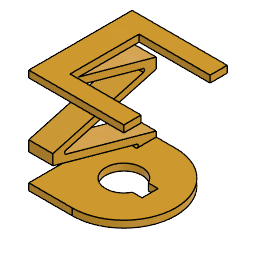
キースイッチ-サンプル (Autodesk Fusion 360 archive; units mm, degrees)
design "ボタン-スプリング"
Autodesk Fusion 360 part; units mm, degrees
note: some values were not read from the file. Set by a fixed rule: which face or edge a step refers to.
sketch "スケッチ1" plane through (0, 0, 0) normal (0, 0, 1) x (1, 0, 0)
  circle A0 centre (0, 0) radius 2.65
  line L0 (0, -7.5) -> (0, 7.5)
  line L1 (0, 7.5) -> (-6.3, 7.5)
  line L2 (-6.3, 7.5) -> (-6.3, -7.5)
  line L3 (-6.3, -7.5) -> (0, -7.5)
  line L4 (0, -7.5) -> (0, 7.5)
  arc A1 (0, -7.5) -> (0, 7.5) centre (0, 0) ccw
  line L5 (2.65, 0) -> (-2.65, 0)
  line L6 (3.8, 1.15) -> (1.5, 1.15)
  line L7 (1.5, 1.15) -> (1.5, -1.15)
  line L8 (1.5, -1.15) -> (3.8, -1.15)
  line L9 (3.8, -1.15) -> (3.8, 1.15)
  line L10 (3.8, 1.15) -> (1.5, -1.15) construction
  line L11 (1.5, 1.15) -> (3.8, -1.15) construction
  point P0 (2.65, 0)
  dimension "d1" = 5.3
  dimension "d2" = 15
  dimension "d5" = 6.3
  dimension "d6" = 15
  dimension "d31" = 2.3
  dimension "d32" = 2.3
  constraint coincident A0.centre A1.centre
  constraint midpoint L0 A0.centre
  constraint vertical L0
  constraint horizontal L1
  constraint vertical L2
  constraint horizontal L3
  constraint vertical L4
  constraint midpoint L5 A0.centre
  constraint coincident A0 L5.end
  constraint perpendicular L0 L5
  constraint horizontal L6
  constraint perpendicular L6 L7
  constraint parallel L6 L8
  constraint parallel L7 L9
  constraint coincident L10 P0
  constraint coincident L11 P0
  constraint coincident P0 L5.start
  measures "d1" diameter of A0
  measures "d2" diameter of A1
  measures "d5" distance of A0.centre L2
  measures "d6" distance of L1 L3
  measures "d31" distance of L7.end L8.end
  measures "d32" distance of L6.end L7.end
extrude "押し出し1" add sketch "スケッチ1" along normal blind 1 contours A0 L0 L4 A1 L6 L8 L9 | A0 L0 L1 L2 L3 L4
sketch "スケッチ2" plane through (-6.3, 0, 0) normal (-1, 0, 0) x (0, -1, 0)
  line L0 (-7.5, 0) -> (7.5, 0)
  line L1 (7.5, 0) -> (7.5, 1)
  line L2 (7.5, 1) -> (-7.5, 1)
  line L3 (-7.5, 1) -> (-7.5, 0)
  line L4 (-7.5, 1) -> (-7.5, 16) construction
  line L5 (7.5, 1) -> (7.5, 16) construction
  line L6 (-7.5, 1) -> (-7.5, 1.7604)
  line L7 (-6.5, 1) -> (-7.5, 1)
  line L8 (-7.5, 1) -> (-7.5, 1.7604)
  line L9 (-4.7298, 1.4909) -> (7.5, 4.8825)
  line L10 (-4.663, 1) -> (10.2045, 1) construction
  line L11 (-7.5, 1.7604) -> (5.6313, 5.4021)
  line L12 (5.6313, 5.8839) -> (-7.5, 9.5255)
  line L13 (-5.6313, 10.045) -> (7.5, 6.4034)
  line L14 (7.5, 6.4034) -> (7.5, 4.8825)
  line L15 (-5.6313, 10.5268) -> (7.5, 14.1685)
  line L16 (-7.5, 11.0463) -> (3.758, 14.1685)
  line L17 (-7.5, 11.0463) -> (-7.5, 9.5255)
  line L18 (7.5, 14.1685) -> (3.758, 14.1685)
  arc A0 (-4.7298, 1.4909) -> (-4.663, 1) centre (-4.663, 1.25) ccw
  arc A1 (5.6313, 5.4021) -> (5.6313, 5.8839) centre (5.5645, 5.643) ccw
  arc A2 (-5.6313, 10.5268) -> (-5.6313, 10.045) centre (-5.5645, 10.2859) ccw
  point P0 (6.5, 5.643)
  point P1 (-6.5, 10.2859)
  dimension "d7" = 15
  dimension "d8" = 15
  dimension "d9" = 15.5
  dimension "d15" = 15.5
  dimension "d16" = 1
  dimension "d17" = 1
  dimension "d18" = 15.5
  dimension "d19" = 15.5
  dimension "d20" = 1
  dimension "d21" = 1
  dimension "d22" = 15.5
  dimension "d23" = 15.5
  dimension "d24" = 1
  dimension "d25" = 1
  dimension "d26" = 0.25
  dimension "d27" = 0.25
  dimension "d28" = 0.25
  constraint coincident L2.end L3.start
  constraint perpendicular L2 L4
  constraint coincident L1.end L2.start
  constraint perpendicular L2 L5
  constraint coincident L4 L6.end
  constraint horizontal L7
  constraint vertical L8
  constraint coincident L2 L7.start
  constraint horizontal L10
  constraint coincident L5 L9.end
  constraint coincident L5 L13.end
  constraint coincident L4 L12.end
  constraint coincident L4 L16.start
  constraint coincident L5 L15.end
  constraint parallel L10 L18
  constraint coincident L7.start L9
  constraint coincident L7.start L10
  constraint tangent L9 A0
  constraint tangent L10 A0
  constraint coincident P0 L11
  constraint coincident P0 L12
  constraint tangent L11 A1
  constraint tangent L12 A1
  constraint coincident P1 L15
  constraint coincident P1 L13
  constraint tangent L15 A2
  constraint tangent L13 A2
  measures "d7" distance of L2.end L4.end
  measures "d8" distance of L1.end L5.end
  measures "d9" angle of L9 L10
  measures "d15" angle of L10 L11
  measures "d16" distance of L9 L11
  measures "d17" distance of L7.start L2.end
  measures "d18" angle of L10 L12
  measures "d19" angle of L10 L13
  measures "d20" distance of L12 L13
  measures "d21" distance of P0 L14
  measures "d22" angle of L10 L15
  measures "d23" angle of L10 L16
  measures "d24" distance of L15 L16
  measures "d25" distance of P1 L17
  measures "d26" radius of A0
  measures "d27" radius of A1
  measures "d28" radius of A2
extrude "押し出し2" add sketch "スケッチ2" against normal blind 3.5 contours L2 L6 L7 L8 L9 L11 L12 L13 L14 L15 L16 L17 L18 A0 A1 A2
sketch "スケッチ3" plane through (0, 0, 14.1685) normal (0, 0, 1) x (-1, 0, 0)
  line L0 (6.3, 3.758) -> (6.3, 7.5)
  line L1 (6.3, 7.5) -> (2.8, 7.5)
  line L2 (2.8, 7.5) -> (2.8, 3.758)
  line L3 (2.8, 3.758) -> (6.3, 3.758)
  line L4 (2.8, -4.663) -> (6.3, -4.663)
  line L5 (6.3, -4.663) -> (6.3, 7.5)
  line L6 (6.3, 7.5) -> (0, 7.5)
  arc A0 (0, 7.5) -> (0, -7.5) centre (0, 0) ccw
  line L7 (0, -7.5) -> (2.8, -7.5)
  line L8 (2.8, -7.5) -> (2.8, -4.663)
  line L9 (-3.8, -1.15) -> (-3.8, 1.15)
  line L10 (-3.8, 1.15) -> (-2.3875, 1.15)
  arc A1 (-2.3875, -1.15) -> (-2.3875, 1.15) centre (0, 0) ccw
  line L11 (-2.3875, -1.15) -> (-3.8, -1.15)
  line L12 (6.3, -7.5) -> (6.3, 3.758)
  line L13 (6.3, 3.758) -> (2.8, 3.758)
  line L14 (2.8, 3.758) -> (2.8, -7.5)
  line L15 (2.8, -7.5) -> (6.3, -7.5)
  line L16 (6.3, 5) -> (6.3, -5)
  line L17 (-7.5, 0) -> (-7.5, -7.5)
  line L18 (-7.5, -7.5) -> (6.3, -7.5)
  line L19 (6.3, -4.663) -> (6.3, -7.5)
  line L20 (6.3, -5) -> (-7.5, -5)
  line L21 (-20, 0) -> (-2.5, 0)
  line L22 (6.3, 5) -> (-7.5, 5)
  line L23 (-7.5, 0) -> (-7.5, 7.5)
  line L24 (6.3, 4.663) -> (6.3, 7.5)
  line L25 (-7.5, 7.5) -> (6.3, 7.5)
  point P0 (6.3, 0)
  dimension "d38" = 5
  constraint midpoint L16 P0
  constraint coincident L12 P0
  constraint coincident L12 L16.end
  constraint midpoint A0 L17.start
  constraint tangent A0 L17
  constraint perpendicular L7 L17
  constraint coincident L12.start L15.end
  constraint perpendicular L12 L18
  constraint coincident L4.end L5.start
  constraint coincident L17 L20.end
  constraint perpendicular L17 L20
  constraint symmetric L17.start L21 L23.start
  constraint symmetric L17.end L21 L23.end
  constraint symmetric L12.start L21 L0.end
  constraint symmetric L4.end L21 L24.start
  constraint symmetric L16.end L21 L16.start
  constraint symmetric L20.end L21 L22.end
  measures "d38" distance of A0.centre L20
extrude "押し出し3" add sketch "スケッチ3" along normal blind 1 contours L0 L2 L3 L5 L13 L16 L22 L24 | L3 L4 L5 L12 L13 L14 L16 | L4 L8 L12 L14 L16 L19 L20 | L0 L1 L2 L5 L6 L22 L24 L25 | L2 L6 A0 L22 L25 | L8 L12 L14 L15 L18 L19 L20 | A0 L22 L23 L25 | A0 L7 L8 L14 L18 L20 | A0 L17 L18 L20
equation "d5 = d1 + 1 mm"
equation "d6 = d2"
equation "d8 = d7"
equation "d15 = d9"
equation "d17 = d16"
equation "d18 = d9"
equation "d19 = d9"
equation "d20 = d16"
equation "d21 = d16"
equation "d22 = d9"
equation "d23 = d9"
equation "d24 = d16"
equation "d25 = d16"
equation "d31 = d32"

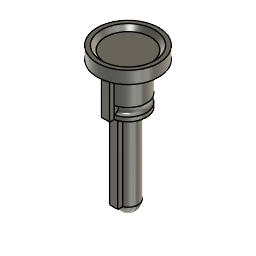
design "ボタンA"
Autodesk Fusion 360 part; units mm, degrees
sketch "スケッチ1" plane through (0, 0, 0) normal (0, 0, 1) x (1, 0, 0)
  circle A0 centre (0, 0) radius 7.5
  dimension "d1" = 15
  constraint coincident A0.centre origin
  measures "d1" diameter of A0
extrude "押し出し1" add sketch "スケッチ1" along normal blind 2
sketch "スケッチ2" plane through (0, 0, 2) normal (0, 0, 1) x (-1, 0, 0)
  circle A0 centre (0, 0) radius 7.5
  circle A1 centre (0, 0) radius 6.5
  dimension "d4" = 13
  constraint coincident A0.centre A1.centre
  measures "d4" diameter of A1
extrude "押し出し2" add sketch "スケッチ2" along normal blind 1
chamfer "面取り1" distance 1 angle 45 1 edges at (6.0601, 2.3505, 2)
sketch "スケッチ3" plane through (0, 0, 0) normal (0, 0, -1) x (1, 0, 0)
  circle A0 centre (0, 0) radius 7.5
  line L0 (0, -2.5) -> (0, 2.5)
  circle A1 centre (0, 0) radius 2.5
  line L1 (1, 1.5) -> (-1, 1.5)
  line L2 (-1, 1.5) -> (-1, 3.5)
  line L3 (-1, 3.5) -> (1, 3.5)
  line L4 (1, 3.5) -> (1, 1.5)
  line L5 (1, 1.5) -> (-1, 3.5) construction
  line L6 (-1, 1.5) -> (1, 3.5) construction
  circle A2 centre (0, 0) radius 4.5
  line L7 (0.9923, 5.5) -> (-1.0077, 5.5)
  line L8 (-1.0077, 5.5) -> (-1.0077, 3.5)
  line L9 (-1.0077, 3.5) -> (0.9923, 3.5)
  line L10 (0.9923, 3.5) -> (0.9923, 5.5)
  line L11 (0.9923, 5.5) -> (-1.0077, 3.5) construction
  line L12 (-1.0077, 5.5) -> (0.9923, 3.5) construction
  point P0 (0, 2.5)
  point P1 (0, 2.5)
  point P2 (-0.0077, 4.5)
  dimension "d8" = 5
  dimension "d15" = 2.5
  dimension "d22" = 2
  dimension "d23" = 2
  dimension "d24" = 9
  dimension "d25" = 2
  dimension "d26" = 2
  constraint coincident A0.centre A1.centre
  constraint midpoint L0 A0.centre
  constraint vertical L0
  constraint coincident P1 P0
  constraint horizontal L1
  constraint perpendicular L1 L2
  constraint parallel L1 L3
  constraint parallel L2 L4
  constraint coincident L5 P1
  constraint coincident L6 P1
  constraint horizontal L7
  constraint perpendicular L7 L8
  constraint parallel L7 L9
  constraint parallel L8 L10
  constraint coincident L11 P2
  constraint coincident L12 P2
  constraint coincident A2 P2
  measures "d8" diameter of A1
  measures "d15" distance of A0.centre P1
  measures "d22" distance of L2.end L3.end
  measures "d23" distance of L1.end L2.end
  measures "d24" diameter of A2
  measures "d25" distance of L7.end L8.end
  measures "d26" distance of L7.start L7.end
extrude "押し出し3" add sketch "スケッチ3" along normal blind 29.45 contours L0 A1 L1 L2 | L0 A1 L1 L4 | L0 A1 L1 L2 | L0 A1 L1 L4 | A1 L2 L3 L4 L9
sketch "スケッチ5" plane through (0, 0, 0) normal (0, 0, -1) x (1, 0, 0)
  line L0 (-1, 2.2913) -> (-1, 3.5)
  line L1 (-1, 3.5) -> (0.9923, 3.5)
  line L2 (1, 3.5) -> (1, 2.2913)
  arc A0 (-1, 2.2913) -> (1, 2.2913) centre (0, 0) ccw
  circle A1 centre (0, 0) radius 7.5
  line L3 (0.9923, 3.5) -> (1, 3.5)
extrude "押し出し4" add sketch "スケッチ3" along normal blind 10 contours A1 L2 L3 L4 A2 L8 L9 L10 | L3 A2 L8 L9 L10 | A2 L7 L8 L10
sphere "球プリミティブ1" add diameter 5 placed x (1, 0, 0) y (0, -1, 0) z (0, 0, -1) at (0, 0, -29.45)
ref_plane "作業平面1" through (0, 0, -8) normal (0, 0, 1) x (-1, 0, 0)
sketch "スケッチ7" plane through (0, 0, -8) normal (0, 0, 1) x (1, 0, 0)
  circle A0 centre (0, 0) radius 4.5
  arc A1 (0.9923, -4.3892) -> (-1.0077, -4.3857) centre (0, 0) ccw
  line L0 (0.9923, -4.3892) -> (0.9923, -5.5)
  line L1 (0.9923, -5.5) -> (-1.0077, -5.5)
  line L2 (-1.0077, -5.5) -> (-1.0077, -4.3857)
  line L3 (0.9923, -3.5) -> (1, -3.5)
  line L4 (1, -3.5) -> (1, -2.2913)
  arc A2 (1, -2.2913) -> (-1, -2.2913) centre (0, 0) ccw
  line L5 (-1, -2.2913) -> (-1, -3.5)
  line L6 (-1, -3.5) -> (0.9923, -3.5)
  line L7 (-1.0077, -5.5) -> (1, -5.5)
  line L8 (1, -5.5) -> (1, -3.5)
  line L9 (1, -3.5) -> (-1.0077, -3.5)
  line L10 (-1.0077, -3.5) -> (-1.0077, -5.5)
  line L11 (1, -2.2913) -> (-1, -2.2913)
  line L12 (-1, -2.2913) -> (-1, -3.5)
  line L13 (-1, -3.5) -> (1, -3.5)
  line L14 (1, -3.5) -> (1, -2.2913)
  dimension "d31" = 9
  constraint coincident A0.centre A1.centre
  constraint horizontal L7
  constraint vertical L8
  constraint horizontal L9
  constraint vertical L10
  constraint coincident L3.end L4.start
  constraint coincident L1.end L2.start
  constraint horizontal L11
  constraint vertical L12
  constraint horizontal L13
  constraint vertical L14
  constraint coincident L5.end L6.start
  constraint coincident L4.end A2.start
  measures "d31" diameter of A0
torus "トーラス プリミティブ1" cut centre line diameter 9 section diameter 2 placed x (1, 0, 0) y (0, 1, 0) z (0, 0, 1) at (0, 0, -8)
extrude "押し出し5" add sketch "スケッチ7" along normal blind 2 and the other way blind 1.9 contours A0 A1 L3 L6 L8 L9 L10 L13 | A0 L0 L1 L2 L7 L10 | L3 L4 L5 L6 L9 L11 L12 L13 L14
equation "d9 = 26 mm + 3.45 mm"
equation "d24 = d8 + 4 mm"

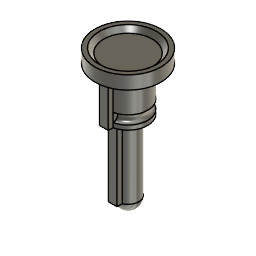
design "ボタンC"
Autodesk Fusion 360 part; units mm, degrees
sketch "スケッチ1" plane through (0, 0, 0) normal (0, 0, 1) x (1, 0, 0)
  circle A0 centre (0, 0) radius 7.5
  dimension "d1" = 15
  constraint coincident A0.centre origin
  measures "d1" diameter of A0
extrude "押し出し1" add sketch "スケッチ1" along normal blind 2
sketch "スケッチ2" plane through (0, 0, 2) normal (0, 0, 1) x (-1, 0, 0)
  circle A0 centre (0, 0) radius 7.5
  circle A1 centre (0, 0) radius 6.5
  dimension "d4" = 13
  constraint coincident A0.centre A1.centre
  measures "d4" diameter of A1
extrude "押し出し2" add sketch "スケッチ2" along normal blind 1
chamfer "面取り1" distance 1 angle 45 1 edges at (6.0601, 2.3505, 2)
sketch "スケッチ3" plane through (0, 0, 0) normal (0, 0, -1) x (1, 0, 0)
  circle A0 centre (0, 0) radius 7.5
  line L0 (0, -2.5) -> (0, 2.5)
  circle A1 centre (0, 0) radius 2.5
  line L1 (1, 1.5) -> (-1, 1.5)
  line L2 (-1, 1.5) -> (-1, 3.5)
  line L3 (-1, 3.5) -> (1, 3.5)
  line L4 (1, 3.5) -> (1, 1.5)
  line L5 (1, 1.5) -> (-1, 3.5) construction
  line L6 (-1, 1.5) -> (1, 3.5) construction
  circle A2 centre (0, 0) radius 4.5
  line L7 (0.9923, 5.5) -> (-1.0077, 5.5)
  line L8 (-1.0077, 5.5) -> (-1.0077, 3.5)
  line L9 (-1.0077, 3.5) -> (0.9923, 3.5)
  line L10 (0.9923, 3.5) -> (0.9923, 5.5)
  line L11 (0.9923, 5.5) -> (-1.0077, 3.5) construction
  line L12 (-1.0077, 5.5) -> (0.9923, 3.5) construction
  point P0 (0, 2.5)
  point P1 (0, 2.5)
  point P2 (-0.0077, 4.5)
  dimension "d8" = 5
  dimension "d15" = 2.5
  dimension "d22" = 2
  dimension "d23" = 2
  dimension "d24" = 9
  dimension "d25" = 2
  dimension "d26" = 2
  constraint coincident A0.centre A1.centre
  constraint midpoint L0 A0.centre
  constraint vertical L0
  constraint coincident P1 P0
  constraint horizontal L1
  constraint perpendicular L1 L2
  constraint parallel L1 L3
  constraint parallel L2 L4
  constraint coincident L5 P1
  constraint coincident L6 P1
  constraint horizontal L7
  constraint perpendicular L7 L8
  constraint parallel L7 L9
  constraint parallel L8 L10
  constraint coincident L11 P2
  constraint coincident L12 P2
  constraint coincident A2 P2
  measures "d8" diameter of A1
  measures "d15" distance of A0.centre P1
  measures "d22" distance of L2.end L3.end
  measures "d23" distance of L1.end L2.end
  measures "d24" diameter of A2
  measures "d25" distance of L7.end L8.end
  measures "d26" distance of L7.start L7.end
extrude "押し出し3" add sketch "スケッチ3" along normal blind 26 contours L0 A1 L1 L2 | L0 A1 L1 L4 | L0 A1 L1 L2 | L0 A1 L1 L4 | A1 L2 L3 L4 L9
sketch "スケッチ5" plane through (0, 0, 0) normal (0, 0, -1) x (1, 0, 0)
  line L0 (-1, 2.2913) -> (-1, 3.5)
  line L1 (-1, 3.5) -> (0.9923, 3.5)
  line L2 (1, 3.5) -> (1, 2.2913)
  arc A0 (-1, 2.2913) -> (1, 2.2913) centre (0, 0) ccw
  circle A1 centre (0, 0) radius 7.5
  line L3 (0.9923, 3.5) -> (1, 3.5)
extrude "押し出し4" add sketch "スケッチ3" along normal blind 10 contours A1 L2 L3 L4 A2 L8 L9 L10 | L3 A2 L8 L9 L10 | A2 L7 L8 L10
sphere "球プリミティブ1" add diameter 5 placed x (1, 0, 0) y (0, -1, 0) z (0, 0, -1) at (0, 0, -26)
ref_plane "作業平面1" through (0, 0, -8) normal (0, 0, 1) x (-1, 0, 0)
sketch "スケッチ7" plane through (0, 0, -8) normal (0, 0, 1) x (1, 0, 0)
  circle A0 centre (0, 0) radius 4.5
  arc A1 (0.9923, -4.3892) -> (-1.0077, -4.3857) centre (0, 0) ccw
  line L0 (0.9923, -4.3892) -> (0.9923, -5.5)
  line L1 (0.9923, -5.5) -> (-1.0077, -5.5)
  line L2 (-1.0077, -5.5) -> (-1.0077, -4.3857)
  line L3 (0.9923, -3.5) -> (1, -3.5)
  line L4 (1, -3.5) -> (1, -2.2913)
  arc A2 (1, -2.2913) -> (-1, -2.2913) centre (0, 0) ccw
  line L5 (-1, -2.2913) -> (-1, -3.5)
  line L6 (-1, -3.5) -> (0.9923, -3.5)
  line L7 (-1.0077, -5.5) -> (1, -5.5)
  line L8 (1, -5.5) -> (1, -3.5)
  line L9 (1, -3.5) -> (-1.0077, -3.5)
  line L10 (-1.0077, -3.5) -> (-1.0077, -5.5)
  line L11 (1, -2.2913) -> (-1, -2.2913)
  line L12 (-1, -2.2913) -> (-1, -3.5)
  line L13 (-1, -3.5) -> (1, -3.5)
  line L14 (1, -3.5) -> (1, -2.2913)
  dimension "d31" = 9
  constraint coincident A0.centre A1.centre
  constraint horizontal L7
  constraint vertical L8
  constraint horizontal L9
  constraint vertical L10
  constraint coincident L3.end L4.start
  constraint coincident L1.end L2.start
  constraint horizontal L11
  constraint vertical L12
  constraint horizontal L13
  constraint vertical L14
  constraint coincident L5.end L6.start
  constraint coincident L4.end A2.start
  measures "d31" diameter of A0
torus "トーラス プリミティブ1" cut centre line diameter 9 section diameter 2 placed x (1, 0, 0) y (0, 1, 0) z (0, 0, 1) at (0, 0, -8)
extrude "押し出し5" add sketch "スケッチ7" along normal blind 2 and the other way blind 1.9 contours A0 A1 L3 L6 L8 L9 L10 L13 | A0 L0 L1 L2 L7 L10 | L3 L4 L5 L6 L9 L11 L12 L13 L14
equation "d24 = d8 + 4 mm"

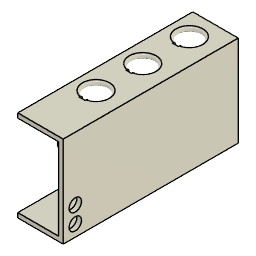
design "キースイッチ-サンプル土台"
Autodesk Fusion 360 part; units mm, degrees
sketch "スケッチ2" plane through (0, 0, 0) normal (0, 0, 1) x (1, 0, 0)
  line L0 (9, -65.0568) -> (9, 9.9432)
  line L1 (9, 9.9432) -> (-8.5, 9.9432)
  line L2 (-8.5, 9.9432) -> (-8.5, -65.0568)
  circle A0 centre (0, 0) radius 4.75
  line L3 (0, -4.75) -> (0, 4.75)
  line L4 (-1.25, -6) -> (1.25, -6)
  line L5 (1.25, -6) -> (1.25, -3.5)
  line L6 (1.25, -3.5) -> (-1.25, -3.5)
  line L7 (-1.25, -3.5) -> (-1.25, -6)
  line L8 (-1.25, -6) -> (1.25, -3.5) construction
  line L9 (1.25, -6) -> (-1.25, -3.5) construction
  line L10 (1.25, -23.5) -> (-1.25, -23.5)
  line L11 (1.25, -26) -> (1.25, -23.5)
  line L12 (0, -24.75) -> (0, -15.25)
  line L13 (-1.25, -26) -> (1.25, -26)
  line L14 (1.25, -26) -> (-1.25, -23.5) construction
  line L15 (-1.25, -23.5) -> (-1.25, -26)
  line L16 (-1.25, -26) -> (1.25, -23.5) construction
  circle A1 centre (0, -20) radius 4.75
  line L17 (1.25, -46) -> (-1.25, -43.5) construction
  line L18 (-1.25, -43.5) -> (-1.25, -46)
  line L19 (-1.25, -46) -> (1.25, -46)
  line L20 (0, -44.75) -> (0, -35.25)
  line L21 (1.25, -46) -> (1.25, -43.5)
  line L22 (1.25, -43.5) -> (-1.25, -43.5)
  circle A2 centre (0, -40) radius 4.75
  line L23 (-1.25, -46) -> (1.25, -43.5) construction
  line L24 (9, -65.0568) -> (-8.5, -65.0568)
  point P0 (0, -4.75)
  point P1 (0, -20)
  point P2 (0, -20)
  point P3 (0, -24.75)
  point P4 (0, -44.75)
  point P5 (0, -40)
  point P6 (0, -40)
  dimension "d4" = 9.5
  dimension "d5" = 2.5
  dimension "d6" = 2.5
  dimension "d16" = 9
  dimension "d17" = 8.5
  dimension "d48" = 9.5
  dimension "d49" = 2.5
  dimension "d50" = 2.5
  dimension "d51" = 20
  dimension "d55" = 9.5
  dimension "d56" = 2.5
  dimension "d57" = 2.5
  dimension "d61" = 20
  dimension "d108" = 75
  constraint parallel L0 L2
  constraint coincident A0.centre origin
  constraint coincident A0 P0
  constraint coincident A0 L3.end
  constraint vertical L3
  constraint horizontal L4
  constraint perpendicular L4 L5
  constraint parallel L4 L6
  constraint parallel L5 L7
  constraint coincident L8 P0
  constraint coincident L9 P0
  constraint coincident P0 L3.start
  constraint vertical A0.centre P0
  constraint coincident P2 P1
  constraint coincident P3 A1
  constraint coincident L12.end A1
  constraint vertical L12
  constraint horizontal L13
  constraint perpendicular L11 L13
  constraint parallel L10 L13
  constraint parallel L11 L15
  constraint coincident P3 L16
  constraint coincident P3 L14
  constraint coincident P3 L12.start
  constraint vertical P3 P2
  constraint coincident P6 P5
  constraint coincident P4 A2
  constraint coincident L20.end A2
  constraint vertical L20
  constraint horizontal L19
  constraint perpendicular L19 L21
  constraint parallel L19 L22
  constraint parallel L18 L21
  constraint coincident P4 L23
  constraint coincident P4 L17
  constraint coincident P4 L20.start
  constraint vertical P4 P6
  constraint vertical A0.centre P5
  constraint vertical A0.centre P2
  constraint horizontal L24
  constraint coincident L2.end L24.end
  constraint perpendicular L1 L2
  constraint perpendicular L2 L24
  measures "d4" diameter of A0
  measures "d5" distance of L5.end L6.end
  measures "d6" distance of L4.end L5.end
  measures "d16" distance of L0 A0.centre
  measures "d17" distance of L2 A0.centre
  measures "d48" diameter of A1
  measures "d49" distance of L10.start L10.end
  measures "d50" distance of L11.start L10.start
  measures "d51" distance of A0.centre P2
  measures "d55" diameter of A2
  measures "d56" distance of L21.end L17.end
  measures "d57" distance of L21.end L17.start
  measures "d61" distance of P2 P6
  measures "d108" distance of L0.start L0.end
extrude "押し出し2" add sketch "スケッチ2" along normal blind 2
sketch "スケッチ3" plane through (9, 0, 0) normal (1, 0, 0) x (0, 1, 0)
  line L0 (-65.0568, 0) -> (9.9432, 0)
  line L1 (9.9432, 0) -> (9.9432, 2)
  line L2 (9.9432, 2) -> (-65.0568, 2)
  line L3 (-65.0568, 2) -> (9.9432, 2)
  line L4 (9.9432, 2) -> (9.9432, -37)
  line L5 (9.9432, -37) -> (-65.0568, -37)
  line L6 (-65.0568, -37) -> (-65.0568, 2)
  line L7 (-65.0568, 2) -> (-65.0568, 0)
  point P0 (9.9432, 2)
  dimension "d11" = 39
  constraint horizontal L3
  constraint vertical L4
  constraint horizontal L5
  constraint vertical L6
  constraint coincident L2.end L3.start
  constraint coincident P0 L1.end
  measures "d11" distance of P0 L4.end
extrude "押し出し3" add sketch "スケッチ3" along normal blind 2
sketch "スケッチ4" plane through (9, 0, 0) normal (-1, 0, 0) x (0, -1, 0)
  line L0 (65.0568, 0) -> (-9.9432, 0)
  line L1 (-9.9432, 0) -> (-9.9432, -37)
  line L2 (-9.9432, -37) -> (65.0568, -37)
  line L3 (65.0568, -37) -> (65.0568, 0)
  line L4 (-9.9432, 0) -> (65.0568, 0)
  line L5 (-9.9432, -37) -> (65.0568, -37)
  line L6 (65.0568, -37) -> (65.0568, -35)
  line L7 (65.0568, -35) -> (-9.9432, -35)
  line L8 (-9.9432, -35) -> (-9.9432, -37)
  line L9 (48.0568, 0) -> (50.0568, 0)
  line L10 (48.0568, -17) -> (-9.9432, -17)
  line L11 (-9.9432, -17) -> (-9.9432, -19)
  line L12 (-9.9432, -19) -> (48.0568, -19)
  line L13 (48.0568, -17) -> (48.0568, -19)
  dimension "d47" = 2
  dimension "d111" = 2
  dimension "d112" = 17
  dimension "d135" = 58
  constraint horizontal L5
  constraint vertical L6
  constraint horizontal L7
  constraint vertical L8
  constraint coincident L3 L6.end
  constraint coincident L1.end L2.start
  constraint horizontal L9
  constraint coincident L0 L9.start
  constraint horizontal L10
  constraint vertical L11
  constraint horizontal L12
  constraint coincident L1 L11.end
  constraint perpendicular L12 L13
  constraint coincident L10.start L13.start
  measures "d47" distance of L2.end L6.end
  measures "d111" distance of L10 L12
  measures "d112" distance of L4 L10
  measures "d135" distance of L1 L13
extrude "押し出し4" add sketch "スケッチ4" along normal blind 17.5 contours L1 L2 L3 L5 L6 L7 L8 | L1 L10 L11 L12 L13
sketch "スケッチ5" plane through (0, 0, -17) normal (0, 0, 1) x (-1, 0, 0)
  line L0 (8.5, -9.9432) -> (8.5, 48.0568)
  line L1 (-9, 65.0568) -> (-9, 50.0568)
  line L2 (-9, -9.9432) -> (8.5, -9.9432)
  circle A0 centre (0, 0) radius 2.65
  line L3 (0, 2.65) -> (0, -2.65)
  line L4 (1.15, 4) -> (1.15, 1.5)
  line L5 (1.15, 1.5) -> (-1.15, 1.5)
  line L6 (-1.15, 1.5) -> (-1.15, 4)
  line L7 (3, 7) -> (-3, 7)
  line L8 (-3, 7) -> (-3, 4)
  line L9 (-3, 4) -> (3, 4)
  line L10 (3, 4) -> (3, 7)
  line L11 (3, 7) -> (-3, 4) construction
  line L12 (-3, 7) -> (3, 4) construction
  circle A1 centre (0, 20) radius 2.65
  line L13 (-3, 27) -> (3, 24) construction
  line L14 (-1.15, 21.5) -> (-1.15, 24)
  line L15 (0, 22.65) -> (0, 17.35)
  line L16 (-3, 27) -> (-3, 24)
  line L17 (1.15, 21.5) -> (-1.15, 21.5)
  line L18 (1.15, 24) -> (1.15, 21.5)
  line L19 (-3, 24) -> (3, 24)
  line L20 (3, 27) -> (-3, 24) construction
  line L21 (3, 24) -> (3, 27)
  line L22 (3, 27) -> (-3, 27)
  line L23 (-1.15, 41.5) -> (-1.15, 44)
  line L24 (1.15, 44) -> (1.15, 41.5)
  line L25 (-3, 47) -> (-3, 44)
  line L26 (1.15, 41.5) -> (-1.15, 41.5)
  line L27 (-3, 47) -> (3, 44) construction
  line L28 (3, 47) -> (-3, 44) construction
  line L29 (3, 47) -> (-3, 47)
  line L30 (0, 42.65) -> (0, 37.35)
  circle A2 centre (0, 40) radius 2.65
  line L31 (-3, 44) -> (3, 44)
  line L32 (3, 44) -> (3, 47)
  line L33 (-9, 50.0568) -> (8.5, 50.0568)
  line L34 (-9, 48.0568) -> (-9, -9.9432)
  line L35 (8.5, 48.0568) -> (-9, 48.0568)
  line L36 (-9, 48.0568) -> (-9, -9.9432)
  line L37 (-9, -9.9432) -> (8.5, -9.9432)
  line L38 (8.5, -9.9432) -> (8.5, 48.0568)
  line L39 (8.5, 48.0568) -> (-9, 48.0568)
  line L40 (-9, 48.0568) -> (-9, -9.9432)
  line L41 (-9, -9.9432) -> (8.5, -9.9432)
  line L42 (8.5, -9.9432) -> (8.5, 48.0568)
  line L43 (8.5, -9.9432) -> (-9, -9.9432)
  line L44 (-9, -9.9432) -> (-9, -6.4432)
  line L45 (-9, -6.4432) -> (8.5, -6.4432)
  line L46 (8.5, -6.4432) -> (8.5, -9.9432)
  line L47 (8.5, 13.5568) -> (-9, 13.5568)
  line L48 (-9, 13.5568) -> (-9, 11.5568)
  line L49 (-9, 11.5568) -> (8.5, 11.5568)
  line L50 (8.5, 11.5568) -> (8.5, 13.5568)
  line L51 (8.5, 33.5568) -> (-9, 33.5568)
  line L52 (-9, 33.5568) -> (-9, 31.5568)
  line L53 (-9, 31.5568) -> (8.5, 31.5568)
  line L54 (8.5, 31.5568) -> (8.5, 33.5568)
  line L55 (8.5, 48.0568) -> (-9, 48.0568)
  point P0 (0, 2.65)
  point P1 (0, 5.5)
  point P2 (0, 20)
  point P3 (0, 20)
  point P4 (0, 22.65)
  point P5 (0, 25.5)
  point P6 (0, 40)
  point P7 (0, 42.65)
  point P8 (0, 45.5)
  point P9 (0, 40)
  dimension "d22" = 5.3
  dimension "d23" = 2.3
  dimension "d87" = 6
  dimension "d88" = 3
  dimension "d89" = 5.5
  dimension "d90" = 1.5
  dimension "d91" = 2.3
  dimension "d92" = 5.3
  dimension "d93" = 2.3
  dimension "d94" = 6
  dimension "d95" = 3
  dimension "d96" = 5.5
  dimension "d97" = 1.5
  dimension "d98" = 2.3
  dimension "d99" = 20
  dimension "d100" = 5.3
  dimension "d101" = 2.3
  dimension "d102" = 6
  dimension "d103" = 3
  dimension "d104" = 5.5
  dimension "d105" = 1.5
  dimension "d106" = 2.3
  dimension "d107" = 20
  dimension "d116" = 3.5
  dimension "d117" = 20
  dimension "d118" = 2
  dimension "d119" = 20
  dimension "d120" = 2
  constraint coincident A0.centre origin
  constraint midpoint L3 A0.centre
  constraint coincident A0 L3.end
  constraint parallel L0 L3
  constraint parallel L4 L6
  constraint coincident P0 L3.start
  constraint horizontal L7
  constraint perpendicular L7 L8
  constraint parallel L7 L9
  constraint parallel L8 L10
  constraint coincident L11 P1
  constraint coincident L12 P1
  constraint coincident L4.start L9
  constraint perpendicular L4 L9
  constraint coincident L6.end L9
  constraint perpendicular L3 L5
  constraint coincident P3 P2
  constraint midpoint P3 L15
  constraint coincident L15.end A1
  constraint parallel L14 L18
  constraint coincident P4 L15.start
  constraint horizontal L22
  constraint perpendicular L16 L22
  constraint parallel L19 L22
  constraint parallel L16 L21
  constraint coincident P5 L20
  constraint coincident P5 L13
  constraint coincident L18.start L19
  constraint perpendicular L18 L19
  constraint coincident L14.end L19
  constraint perpendicular L15 L17
  constraint coincident P9 P6
  constraint midpoint P9 L30
  constraint coincident L30.end A2
  constraint parallel L23 L24
  constraint coincident P7 L30.start
  constraint horizontal L29
  constraint perpendicular L25 L29
  constraint parallel L29 L31
  constraint parallel L25 L32
  constraint coincident P8 L28
  constraint coincident P8 L27
  constraint coincident L24.start L31
  constraint perpendicular L24 L31
  constraint coincident L23.end L31
  constraint perpendicular L26 L30
  constraint vertical A0.centre P3
  constraint vertical A0.centre P9
  constraint vertical P5 P8
  constraint horizontal L43
  constraint vertical L44
  constraint horizontal L45
  constraint vertical L46
  constraint coincident L0.start L2.end
  constraint horizontal L47
  constraint vertical L48
  constraint horizontal L49
  constraint vertical L50
  constraint coincident L40 L48.end
  constraint coincident L0 L47.start
  constraint horizontal L51
  constraint vertical L52
  constraint horizontal L53
  constraint vertical L54
  constraint coincident L40 L52.end
  constraint coincident L38 L51.start
  measures "d22" diameter of A0
  measures "d23" distance of L4.end L5.end
  measures "d87" distance of L8.end L9.end
  measures "d88" distance of L7.end L8.end
  measures "d89" distance of A0.centre P1
  measures "d90" distance of A0.centre L5
  measures "d92" diameter of A1
  measures "d93" distance of L17.start L14.start
  measures "d94" distance of L16.end L13.end
  measures "d95" distance of L13.start L16.end
  measures "d96" distance of P3 P5
  measures "d97" distance of P3 L17
  measures "d99" distance of A0.centre P3
  measures "d100" diameter of A2
  measures "d101" distance of L23.start L24.end
  measures "d102" distance of L25.end L27.end
  measures "d103" distance of L25.start L25.end
  measures "d104" distance of P8 P9
  measures "d105" distance of P9 L26
  measures "d107" distance of P3 P9
  measures "d116" distance of L0.start L45.end
  measures "d117" distance of L45 L47
  measures "d118" distance of L47 L49
  measures "d119" distance of L47 L51
  measures "d120" distance of L51 L53
extrude "押し出し14" cut sketch "スケッチ5" along normal blind 2 from surface at -2 contours A0 L3 L4 L5 | A0 L3 L5 L6 | A0 L4 L6 L9 | A0 L3 L5 L6 | A0 L3 L4 L5 | L7 L8 L9 L10 | A1 L15 L17 L18 | A1 L14 L15 L17 | A1 L14 L18 L19 | A1 L14 L15 L17 | A1 L15 L17 L18 | L16 L19 L21 L22 | L23 L26 L30 A2 | L23 L26 L30 A2 | L23 L24 A2 L31 | L24 L26 L30 A2 | L24 L26 L30 A2 | L25 L29 L31 L32
extrude "押し出し15" add sketch "スケッチ5" along normal blind 1 contours L0 L2 L34 L36 L37 L38 L40 L41 L42 L43 L44 L45 L46 | L0 L34 L36 L38 L40 L42 L47 L48 L49 L50 | L0 L34 L36 L38 L40 L42 L51 L52 L53 L54
fillet "フィレット1" radius 1 12 edges at (0, 2.65, -17) (0, -17.35, -17) (0, -37.35, -17) (0, 4.75, 2) (0, -15.25, 2) (0, -35.25, 2) (0, -35.25, 0) (0, -15.25, 0) (0, 4.75, 0) (0, 2.65, -19) (0, -17.35, -19) (0, -37.35, -19)
sketch "スケッチ11" plane through (9, 0, 0) normal (-1, 0, 0) x (0, -1, 0)
  circle A0 centre (59.8875, -25) radius 2.5
  spline S0 degree 3 poles (43.4641, -17) (43.3309, -17) (43.1738, -17.0302) (42.9274, -17.128) (42.7936, -17.2125) (42.606, -17.3902) (42.5173, -17.5135) (42.4179, -17.7392) (42.3875, -17.88) (42.3875, -18) knots 0.151292 0.151292 0.151292 0.151292 0.191268 0.191268 0.230832 0.230832 0.268794 0.268794 0.304806 0.304806 0.304806 0.304806
  line L0 (36.35, -19) -> (43.4641, -19)
  spline S1 degree 3 poles (42.3875, -18) (42.3875, -17.88) (42.4179, -17.7392) (42.5173, -17.5135) (42.606, -17.3902) (42.7936, -17.2125) (42.9274, -17.128) (43.1738, -17.0302) (43.3309, -17) (43.4641, -17) knots 0.304806 0.304806 0.304806 0.304806 0.340818 0.340818 0.37878 0.37878 0.418344 0.418344 0.45832 0.45832 0.45832 0.45832
  line L1 (37.3875, -17) -> (42.3875, -17)
  line L2 (42.3875, -17) -> (42.3875, -18)
  line L3 (42.3875, -18) -> (37.3875, -18)
  line L4 (37.3875, -18) -> (37.3875, -17)
  line L5 (39.8875, -21.7117) -> (39.8875, -12.2883)
  circle A1 centre (59.8875, -32) radius 2.5
  line L6 (43.4641, -17) -> (36.35, -17)
  spline S2 degree 3 poles (42.3875, -18) (42.3875, -18.12) (42.4179, -18.2608) (42.5173, -18.4865) (42.606, -18.6098) (42.7936, -18.7875) (42.9274, -18.872) (43.1738, -18.9698) (43.3309, -19) (43.4641, -19) knots 0.304806 0.304806 0.304806 0.304806 0.340818 0.340818 0.37878 0.37878 0.418344 0.418344 0.45832 0.45832 0.45832 0.45832
  spline S3 degree 3 poles (43.4641, -19) (43.3309, -19) (43.1738, -18.9698) (42.9274, -18.872) (42.7936, -18.7875) (42.606, -18.6098) (42.5173, -18.4865) (42.4179, -18.2608) (42.3875, -18.12) (42.3875, -18) knots 0.151292 0.151292 0.151292 0.151292 0.191268 0.191268 0.230832 0.230832 0.268794 0.268794 0.304806 0.304806 0.304806 0.304806
  point P0 (39.8875, -17)
  dimension "d125" = 5
  dimension "d126" = 20
  dimension "d127" = 6
  dimension "d131" = 5
  dimension "d132" = 5
  dimension "d133" = 7
  constraint horizontal L1
  constraint vertical L2
  constraint horizontal L3
  constraint vertical L4
  constraint coincident S0.end S1.start
  constraint midpoint L5 P0
  constraint coincident L1 P0
  constraint perpendicular L1 L5
  constraint midpoint L1 L5
  constraint vertical A0.centre A1.centre
  measures "d125" diameter of A0
  measures "d126" distance of A0.centre L5
  measures "d127" distance of A0.centre L0
  measures "d132" diameter of A1
  measures "d133" vertical distance of A0.centre A1.centre
extrude "押し出し16" cut sketch "スケッチ11" against normal blind 2 contours A0 | A1
move_face "面をオフセット1" offset -0.15 2 faces at (9.6667, -62.375, -25.2489) (10.3333, -58.5311, -34.1001)
equation "d19 = 2 mm"
equation "d47 = d19"
equation "d61 = d51"
equation "d107 = d99"
equation "d120 = d118"

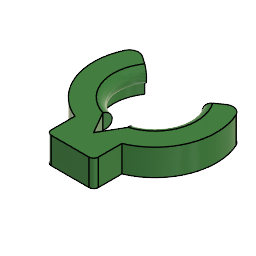
design "ボタンストッパー"
Autodesk Fusion 360 part; units mm, degrees
sketch "スケッチ1" plane through (0, 0, 0) normal (0, 0, 1) x (1, 0, 0)
  circle A0 centre (0, 0) radius 4.5
  line L0 (1, 5.5) -> (-1, 5.5)
  line L1 (-1, 5.5) -> (-1, 3.5)
  line L2 (-1, 3.5) -> (1, 3.5)
  line L3 (1, 3.5) -> (1, 5.5)
  line L4 (1, 5.5) -> (-1, 3.5) construction
  line L5 (-1, 5.5) -> (1, 3.5) construction
  line L6 (-4.5, 0) -> (4.5, 0)
  arc A1 (-5.324488, 3.728247) -> (-6.5, 0) centre (0, 0) ccw
  line L7 (-5.324488, 3.728247) -> (0, 0)
  arc A2 (-6.5, 0) -> (0, -6.5) centre (0, 0) ccw
  line L8 (0, 2.5) -> (0, 20)
  arc A3 (6.5, 0) -> (5.324488, 3.728247) centre (0, 0) ccw
  line L9 (5.324488, 3.728247) -> (0, 0)
  arc A4 (0, -6.5) -> (6.5, 0) centre (0, 0) ccw
  line L10 (-2.5, -6) -> (-2.5, -9)
  line L11 (-2.5, -9) -> (2.5, -9)
  line L12 (2.5, -9) -> (2.5, -6)
  line L13 (0, 9) -> (0, -9)
  line L14 (0, -6.5) -> (-1.258345, -4.320482)
  line L15 (0, -6.5) -> (1.258345, -4.320482)
  point P0 (0, 4.5)
  point P1 (0, -6.5)
  dimension "d1" = 9
  dimension "d2" = 2
  dimension "d3" = 2
  dimension "d5" = 35
  dimension "d6" = 2
  dimension "d9" = 5
  dimension "d17" = 9
  dimension "d18" = 2.5
  dimension "d19" = 90
  dimension "d20" = 30
  constraint coincident A0.centre A1.centre
  constraint horizontal L0
  constraint perpendicular L0 L1
  constraint parallel L0 L2
  constraint parallel L1 L3
  constraint coincident L4 P0
  constraint coincident L5 P0
  constraint coincident A0 P0
  constraint vertical A0.centre P0
  constraint midpoint L6 A0.centre
  constraint coincident A0 L6.end
  constraint horizontal L6
  constraint symmetric A1.end L8 A3.start
  constraint symmetric A1 L8 A3
  constraint symmetric A0.centre L8 A1.centre
  constraint symmetric P1 L8 A2.end
  constraint symmetric A2 L8 A4
  constraint parallel L10 L12
  constraint coincident P1 A2.end
  constraint coincident A4 L12.end
  constraint coincident A2 L10.start
  constraint equal L10 L12
  constraint midpoint L13 A0.centre
  constraint coincident L11 L13.end
  constraint perpendicular L11 L13
  constraint midpoint L11 L13.end
  constraint symmetric P1 L13 A2.end
  measures "d1" diameter of A0
  measures "d2" distance of L1.end L2.end
  measures "d3" distance of L0.end L1.end
  measures "d5" angle of L6 L7
  measures "d6" distance of A0 A1
  measures "d9" distance of L10.end L11.end
  measures "d17" distance of A0.centre L11
  measures "d18" distance of L11 P1
  measures "d19" angle of L6 L13
  measures "d20" angle of L13 L14
extrude "押し出し1" add sketch "スケッチ1" along normal blind 3 contours A0 A1 L7 A2 L14 | A2 L10 L11 L13 | A0 A3 L9 A4 L15 | A4 L11 L12 L13 picked at (-2.57109, -5.222027) picked at (-1.117638, -8.147933) picked at (2.57109, -5.222027) picked at (1.117638, -8.147933)
move_face "面をオフセット1" offset 0.1 4 faces at (4.496269, 0.183209, 1) (4.479554, -0.428478, 2) (-4.494886, -0.214483, 1) (-4.496269, 0.183209, 2)
ref_plane "作業平面1" through (0, -2.722325, 2) normal (0, 0, -1) x (-1, 0, 0)
sketch "スケッチ2" plane through (0, 0, 2) normal (0, 0, -1) x (-1, 0, 0)
  line L0 (2.5, -9) -> (-2.5, -9)
  line L1 (-2.5, -9) -> (-2.5, -6)
  arc A0 (2.5, -6) -> (5.324488, 3.728247) centre (0, 0) ccw
  arc A1 (-3.604269, 2.523736) -> (-1.331554, -4.193682) centre (0, 0) ccw
  arc A2 (1.331554, -4.193682) -> (3.604269, 2.523736) centre (0, 0) ccw
  line L2 (2.5, -6) -> (2.5, -9)
  arc A3 (-5.324488, 3.728247) -> (-2.5, -6) centre (0, 0) ccw
pipe "パイプ1" add diameter 2 path "スケッチ2" along A2
pipe "パイプ2" add diameter 2 path "スケッチ2" along A1
fillet "フィレット1" radius 1 2 edges at (-5.324488, 3.728247, 1.5) (5.324488, 3.728247, 1.5)
fillet "フィレット2" radius 0.5 2 edges at (2.5, -9, 1.5) (-2.5, -9, 1.5)
move_face "面をオフセット2" offset -0.2 2 faces at (-4.187326, 1.179042, 1.001243) (4.054853, 1.57544, 2.998757)

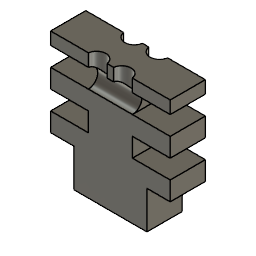
design "スイッチ-ワイヤー保持台"
Autodesk Fusion 360 part; units mm, degrees
sketch "スケッチ1" plane through (0, 0, 0) normal (0, 0, 1) x (1, 0, 0)
  line L0 (3, 1.5) -> (-3, 1.5)
  line L1 (-3, 1.5) -> (-3, -1.5)
  line L2 (-3, -1.5) -> (3, -1.5)
  line L3 (3, -1.5) -> (3, 1.5)
  line L4 (3, 1.5) -> (-3, -1.5) construction
  line L5 (-3, 1.5) -> (3, -1.5) construction
  dimension "d1" = 6
  dimension "d2" = 3
  constraint horizontal L0
  constraint perpendicular L0 L1
  constraint parallel L0 L2
  constraint parallel L1 L3
  constraint coincident L4 origin
  constraint coincident L5 origin
  measures "d1" distance of L1.end L2.end
  measures "d2" distance of L0.end L1.end
extrude "押し出し1" add sketch "スケッチ1" along normal blind 3
sketch "スケッチ2" plane through (0, 0, 3) normal (0, 0, 1) x (-1, 0, 0)
  line L0 (-3, 1.5) -> (-3, -1.5)
  line L1 (-3, -1.5) -> (3, -1.5)
  line L2 (3, -1.5) -> (3, 1.5)
  line L3 (3, 1.5) -> (-3, 1.5)
  line L4 (-4.75, -1.5) -> (4.75, -1.5)
  line L5 (4.75, -1.5) -> (4.75, 1.5)
  line L6 (4.75, 1.5) -> (-4.75, 1.5)
  line L7 (-4.75, 1.5) -> (-4.75, -1.5)
  line L8 (-4.75, -1.5) -> (4.75, 1.5) construction
  line L9 (4.75, -1.5) -> (-4.75, 1.5) construction
  dimension "d5" = 9.5
  dimension "d6" = 3
  constraint horizontal L4
  constraint perpendicular L4 L5
  constraint parallel L4 L6
  constraint parallel L5 L7
  constraint coincident L8 origin
  constraint coincident L9 origin
  measures "d5" distance of L5.end L6.end
  measures "d6" distance of L4.end L5.end
extrude "押し出し2" add sketch "スケッチ2" along normal blind 7
sketch "スケッチ3" plane through (0, 0, 10) normal (0, 0, 1) x (-1, 0, 0)
  line L0 (-4.75, 1.5) -> (-4.75, -1.5)
  line L1 (-4.75, -1.5) -> (4.75, -1.5)
  line L2 (4.75, -1.5) -> (4.75, 1.5)
  line L3 (4.75, 1.5) -> (-4.75, 1.5)
  line L4 (1, 0) -> (-1, 0)
  circle A0 centre (1, 0) radius 0.75 construction
  line L5 (1, 0) -> (2.5, 0)
  circle A1 centre (2.5, 0) radius 0.75 construction
  circle A2 centre (4, 0) radius 0.75 construction
  line L6 (2.5, 0) -> (4, 0)
  circle A3 centre (1, 1.5) radius 0.75
  dimension "d9" = 2
  dimension "d15" = 1.5
  dimension "d17" = 1.5
  dimension "d18" = 1.5
  dimension "d19" = 1.5
  dimension "d20" = 1.5
  dimension "d32" = 1.5
  dimension "d33" = 1
  constraint midpoint L4 origin
  constraint perpendicular L2 L4
  constraint coincident L4.start A0.centre
  constraint horizontal L5
  constraint coincident L5.end A1.centre
  constraint coincident A2.centre L6.end
  constraint perpendicular L2 L6
  constraint coincident L3 A3.centre
  measures "d9" distance of L4.start L4.end
  measures "d15" diameter of A0
  measures "d17" diameter of A1
  measures "d18" distance of L4.start L5.end
  measures "d19" diameter of A2
  measures "d20" distance of L5.end A2.centre
  measures "d32" diameter of A3
  measures "d33" horizontal distance of origin A3.centre
sketch "スケッチ5" plane through (0, -1.5, 0) normal (0, -1, 0) x (1, 0, 0)
  line L0 (-3, 0) -> (3, 0)
  line L1 (3, 0) -> (3, 3)
  line L2 (3, 3) -> (4.75, 3)
  line L3 (4.75, 3) -> (4.75, 10)
  line L4 (4.75, 10) -> (-4.75, 10)
  line L5 (-4.75, 10) -> (-4.75, 3)
  line L6 (-4.75, 3) -> (-3, 3)
  line L7 (-3, 3) -> (-3, 0)
  line L8 (-4.75, 3) -> (-4.75, 4.5)
  line L9 (-4.75, 4.5) -> (-1.75, 4.5)
  line L10 (-1.75, 4.5) -> (-1.75, 6)
  line L11 (-1.75, 6) -> (-4.75, 6)
  line L12 (-4.75, 6) -> (-4.75, 4.5)
  line L13 (-4.75, 6) -> (-4.75, 7.5)
  line L14 (-4.75, 7.5) -> (-1.75, 7.5)
  line L15 (-1.75, 7.5) -> (-1.75, 9)
  line L16 (-1.75, 9) -> (-4.75, 9)
  line L17 (-4.75, 9) -> (-4.75, 7.5)
  line L18 (0, 1.75) -> (0, 22.5)
  line L19 (4.75, 4.5) -> (1.75, 4.5)
  line L20 (1.75, 4.5) -> (1.75, 6)
  line L21 (1.75, 6) -> (4.75, 6)
  line L22 (1.75, 7.5) -> (1.75, 9)
  line L23 (1.75, 9) -> (4.75, 9)
  line L24 (4.75, 9) -> (4.75, 7.5)
  line L25 (4.75, 7.5) -> (1.75, 7.5)
  dimension "d21" = 1.5
  dimension "d22" = 1.5
  dimension "d23" = 1.5
  dimension "d24" = 1.5
  dimension "d25" = 3
  dimension "d26" = 3
  constraint coincident L5.end L6.start
  constraint perpendicular L4 L8
  constraint horizontal L9
  constraint vertical L10
  constraint horizontal L11
  constraint vertical L12
  constraint perpendicular L11 L13
  constraint horizontal L14
  constraint vertical L15
  constraint horizontal L16
  constraint vertical L17
  constraint symmetric L8.end L18 L19.start
  constraint symmetric L9.end L18 L19.end
  constraint symmetric L10.end L18 L20.end
  constraint symmetric L11.end L18 L21.end
  constraint symmetric L13.end L18 L24.end
  constraint symmetric L14.end L18 L22.start
  constraint symmetric L15.end L18 L22.end
  constraint symmetric L16.end L18 L23.end
  measures "d21" distance of L5.end L8.end
  measures "d22" distance of L8.end L11.end
  measures "d23" distance of L11.end L13.end
  measures "d24" distance of L13.end L16.end
  measures "d25" distance of L8.end L9.end
  measures "d26" distance of L13.end L14.end
extrude "押し出し3" cut sketch "スケッチ5" against normal through all contours L5 L9 L10 L11 L12 | L3 L19 L20 L21 | L5 L14 L15 L16 L17 | L3 L22 L23 L24 L25
move_face "面をオフセット1" offset -0.1 4 faces at (-3, 0.5, 1) (-1, 1.5, 2) (1, -1.5, 2) (3, -0.5, 1)
ref_plane "作業平面1" through (-1, 0, 0) normal (1, 0, 0) x (0, 1, 0)
sketch "スケッチ10" plane through (0, 0, 10) normal (0, 0, 1) x (-1, 0, 0)
  line L0 (-4.75, 1.4) -> (-4.75, -1.4)
  line L1 (-4.75, -1.4) -> (4.75, -1.4)
  line L2 (4.75, -1.4) -> (4.75, 1.4)
  line L3 (4.75, 1.4) -> (-4.75, 1.4)
  circle A0 centre (1, -1.5) radius 0.75
  circle A1 centre (1, 1.5) radius 0.75
  circle A2 centre (-1, 1.5) radius 0.75
  circle A3 centre (-1, -1.5) radius 0.75
  dimension "d48" = 1.5
  dimension "d49" = 1.5
  dimension "d61" = 1.5
  dimension "d62" = 1.5
  dimension "d63" = 2
  dimension "d64" = 3
  dimension "d66" = 1
  dimension "d67" = 1.5
  constraint horizontal A0.centre A3.centre
  constraint vertical A2.centre A3.centre
  constraint vertical A0.centre A1.centre
  constraint horizontal A1.centre A2.centre
  measures "d48" diameter of A0
  measures "d49" diameter of A1
  measures "d61" diameter of A2
  measures "d62" diameter of A3
  measures "d63" distance of A0.centre A3.centre
  measures "d64" distance of A2.centre A3.centre
  measures "d66" horizontal distance of origin A3.centre
  measures "d67" vertical distance of origin A3.centre
extrude "押し出し6" cut sketch "スケッチ10" against normal blind 1.75 contours L3 A2 | L3 A2 | L1 A3 | L1 A3 | L3 A1 | L3 A1 | L1 A0 | L1 A0
sketch "スケッチ12" plane through (0, 0, 0) normal (1, 0, 0) x (0, 1, 0)
  line L0 (1.4, 7.5) -> (1.4, 9)
  line L1 (1.4, 9) -> (-1.4, 9)
  line L2 (-1.4, 9) -> (-1.4, 7.5)
  line L3 (-1.4, 7.5) -> (1.4, 7.5)
  circle A0 centre (1.4, 8.25) radius 0.75
  line L4 (0, 2.5) -> (0, 20)
  circle A1 centre (-1.4, 8.25) radius 0.75
  dimension "d59" = 1.5
  constraint midpoint L0 A0.centre
  constraint symmetric A0 L4 A1
  measures "d59" diameter of A0
extrude "押し出し8" cut sketch "スケッチ12" along normal through all and the other way through all contours L0 A0 | L0 A0 | L2 A1 | L2 A1
equation "d5 = 7 mm + 1.25 * 2 mm"
equation "d12 = 0.1 mm"
equation "d25 = ( 1.5 * 2 ) * 1 mm"
equation "d26 = d25"
equation "d30 = 1 mm + d12 + d12"

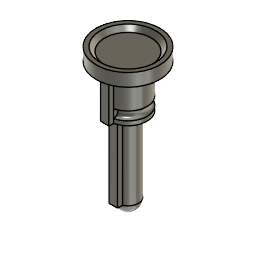
design "ボタンB"
Autodesk Fusion 360 part; units mm, degrees
sketch "スケッチ1" plane through (0, 0, 0) normal (0, 0, 1) x (1, 0, 0)
  circle A0 centre (0, 0) radius 7.5
  dimension "d1" = 15
  constraint coincident A0.centre origin
  measures "d1" diameter of A0
extrude "押し出し1" add sketch "スケッチ1" along normal blind 2
sketch "スケッチ2" plane through (0, 0, 2) normal (0, 0, 1) x (-1, 0, 0)
  circle A0 centre (0, 0) radius 7.5
  circle A1 centre (0, 0) radius 6.5
  dimension "d4" = 13
  constraint coincident A0.centre A1.centre
  measures "d4" diameter of A1
extrude "押し出し2" add sketch "スケッチ2" along normal blind 1
chamfer "面取り1" distance 1 angle 45 1 edges at (6.0601, 2.3505, 2)
sketch "スケッチ3" plane through (0, 0, 0) normal (0, 0, -1) x (1, 0, 0)
  circle A0 centre (0, 0) radius 7.5
  line L0 (0, -2.5) -> (0, 2.5)
  circle A1 centre (0, 0) radius 2.5
  line L1 (1, 1.5) -> (-1, 1.5)
  line L2 (-1, 1.5) -> (-1, 3.5)
  line L3 (-1, 3.5) -> (1, 3.5)
  line L4 (1, 3.5) -> (1, 1.5)
  line L5 (1, 1.5) -> (-1, 3.5) construction
  line L6 (-1, 1.5) -> (1, 3.5) construction
  circle A2 centre (0, 0) radius 4.5
  line L7 (0.9923, 5.5) -> (-1.0077, 5.5)
  line L8 (-1.0077, 5.5) -> (-1.0077, 3.5)
  line L9 (-1.0077, 3.5) -> (0.9923, 3.5)
  line L10 (0.9923, 3.5) -> (0.9923, 5.5)
  line L11 (0.9923, 5.5) -> (-1.0077, 3.5) construction
  line L12 (-1.0077, 5.5) -> (0.9923, 3.5) construction
  point P0 (0, 2.5)
  point P1 (0, 2.5)
  point P2 (-0.0077, 4.5)
  dimension "d8" = 5
  dimension "d15" = 2.5
  dimension "d22" = 2
  dimension "d23" = 2
  dimension "d24" = 9
  dimension "d25" = 2
  dimension "d26" = 2
  constraint coincident A0.centre A1.centre
  constraint midpoint L0 A0.centre
  constraint vertical L0
  constraint coincident P1 P0
  constraint horizontal L1
  constraint perpendicular L1 L2
  constraint parallel L1 L3
  constraint parallel L2 L4
  constraint coincident L5 P1
  constraint coincident L6 P1
  constraint horizontal L7
  constraint perpendicular L7 L8
  constraint parallel L7 L9
  constraint parallel L8 L10
  constraint coincident L11 P2
  constraint coincident L12 P2
  constraint coincident A2 P2
  measures "d8" diameter of A1
  measures "d15" distance of A0.centre P1
  measures "d22" distance of L2.end L3.end
  measures "d23" distance of L1.end L2.end
  measures "d24" diameter of A2
  measures "d25" distance of L7.end L8.end
  measures "d26" distance of L7.start L7.end
extrude "押し出し3" add sketch "スケッチ3" along normal blind 27.75 contours L0 A1 L1 L2 | L0 A1 L1 L4 | L0 A1 L1 L2 | L0 A1 L1 L4 | A1 L2 L3 L4 L9
sketch "スケッチ5" plane through (0, 0, 0) normal (0, 0, -1) x (1, 0, 0)
  line L0 (-1, 2.2913) -> (-1, 3.5)
  line L1 (-1, 3.5) -> (0.9923, 3.5)
  line L2 (1, 3.5) -> (1, 2.2913)
  arc A0 (-1, 2.2913) -> (1, 2.2913) centre (0, 0) ccw
  circle A1 centre (0, 0) radius 7.5
  line L3 (0.9923, 3.5) -> (1, 3.5)
extrude "押し出し4" add sketch "スケッチ3" along normal blind 10 contours A1 L2 L3 L4 A2 L8 L9 L10 | L3 A2 L8 L9 L10 | A2 L7 L8 L10
sphere "球プリミティブ1" add diameter 5 placed x (1, 0, 0) y (0, -1, 0) z (0, 0, -1) at (0, 0, -27.75)
ref_plane "作業平面1" through (0, 0, -8) normal (0, 0, 1) x (-1, 0, 0)
sketch "スケッチ7" plane through (0, 0, -8) normal (0, 0, 1) x (1, 0, 0)
  circle A0 centre (0, 0) radius 4.5
  arc A1 (0.9923, -4.3892) -> (-1.0077, -4.3857) centre (0, 0) ccw
  line L0 (0.9923, -4.3892) -> (0.9923, -5.5)
  line L1 (0.9923, -5.5) -> (-1.0077, -5.5)
  line L2 (-1.0077, -5.5) -> (-1.0077, -4.3857)
  line L3 (0.9923, -3.5) -> (1, -3.5)
  line L4 (1, -3.5) -> (1, -2.2913)
  arc A2 (1, -2.2913) -> (-1, -2.2913) centre (0, 0) ccw
  line L5 (-1, -2.2913) -> (-1, -3.5)
  line L6 (-1, -3.5) -> (0.9923, -3.5)
  line L7 (-1.0077, -5.5) -> (1, -5.5)
  line L8 (1, -5.5) -> (1, -3.5)
  line L9 (1, -3.5) -> (-1.0077, -3.5)
  line L10 (-1.0077, -3.5) -> (-1.0077, -5.5)
  line L11 (1, -2.2913) -> (-1, -2.2913)
  line L12 (-1, -2.2913) -> (-1, -3.5)
  line L13 (-1, -3.5) -> (1, -3.5)
  line L14 (1, -3.5) -> (1, -2.2913)
  dimension "d31" = 9
  constraint coincident A0.centre A1.centre
  constraint horizontal L7
  constraint vertical L8
  constraint horizontal L9
  constraint vertical L10
  constraint coincident L3.end L4.start
  constraint coincident L1.end L2.start
  constraint horizontal L11
  constraint vertical L12
  constraint horizontal L13
  constraint vertical L14
  constraint coincident L5.end L6.start
  constraint coincident L4.end A2.start
  measures "d31" diameter of A0
torus "トーラス プリミティブ1" cut centre line diameter 9 section diameter 2 placed x (1, 0, 0) y (0, 1, 0) z (0, 0, 1) at (0, 0, -8)
extrude "押し出し5" add sketch "スケッチ7" along normal blind 2 and the other way blind 1.9 contours A0 A1 L3 L6 L8 L9 L10 L13 | A0 L0 L1 L2 L7 L10 | L3 L4 L5 L6 L9 L11 L12 L13 L14
equation "d9 = 26 mm + 1.75 mm"
equation "d24 = d8 + 4 mm"
